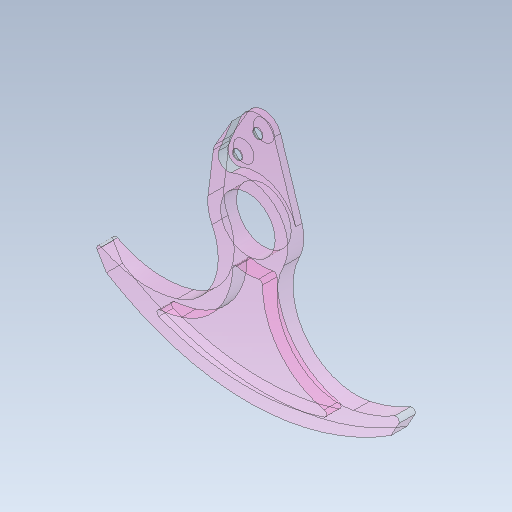
# Autodesk Inventor part: 新型３ヘッケン
Saved by Autodesk Inventor 2020 (Build 240168000, 168)
## iProperties
Created: 2019-03-26
Part Number: 新型３ヘッケン
Material: ポリカーボネート、クリア
Document SubType Name: Modeling
Designer: tanjihayato
Density: 1.2 g/cm^3
Appearance: ポリカーボネート - クリア
Mass: 7.67377 g
Surface Area: 65.6128 cm^2
Volume: 6.39481 cm^3
Author: tanjihayato
Autodesk Inventor part; units mm, degrees
ref_plane "YZ Plane" through (0, 0, 0) normal (1, 0, 0) x (0, 1, 0)
ref_plane "XZ Plane" through (0, 0, 0) normal (0, 1, 0) x (-1, 0, 0)
ref_plane "XY Plane" through (0, 0, 0) normal (0, 0, 1) x (1, 0, 0)
sketch "スケッチ1" plane through (0, 0, 0) normal (0, 0, 1) x (1, 0, 0)
  spline S0 degree 4 poles (44.6679, -57.7205) (44.3779, -57.9011) (43.9715, -58.1517) (43.4481, -58.4698) (42.8069, -58.8523) (42.3406, -59.127) (41.8739, -59.3984) (41.4069, -59.6666) (40.9394, -59.9316) (40.4714, -60.1934) (40.003, -60.452) (39.5341, -60.7075) (39.0646, -60.9598) (38.5946, -61.209) (38.124, -61.455) (37.6528, -61.698) (37.181, -61.9378) (36.7086, -62.1745) (36.2356, -62.4081) (35.7619, -62.6386) (35.2875, -62.8661) (34.8124, -63.0904) (34.3367, -63.3117) (33.8603, -63.5299) (33.3831, -63.745) (32.9053, -63.9571) (32.4267, -64.166) (31.9475, -64.3719) (31.4674, -64.5748) (30.9867, -64.7745) (30.5052, -64.9712) (30.023, -65.1648) (29.54, -65.3554) (29.0563, -65.5428) (28.5719, -65.7272) (28.0867, -65.9085) (27.6008, -66.0867) (27.1141, -66.2618) (26.6267, -66.4339) (26.1386, -66.6028) (25.6497, -66.7686) (25.1602, -66.9313) (24.6699, -67.0909) (24.1789, -67.2474) (23.6872, -67.4008) (23.1948, -67.551) (22.7018, -67.6981) (22.208, -67.8421) (21.7136, -67.983) (21.2185, -68.1207) (20.7227, -68.2552) (20.2264, -68.3866) (19.7293, -68.5148) (19.2317, -68.6399) (18.7335, -68.7617) (18.2346, -68.8805) (17.7352, -68.996) (17.2352, -69.1083) (16.7346, -69.2175) (16.2335, -69.3234) (15.7318, -69.4261) (15.2297, -69.5257) (14.727, -69.622) (14.2238, -69.7151) (13.7202, -69.805) (13.2161, -69.8917) (12.7115, -69.9751) (12.2065, -70.0553) (11.7011, -70.1322) (11.1953, -70.2059) (10.6891, -70.2764) (10.1825, -70.3436) (9.6756, -70.4076) (9.1683, -70.4683) (8.6608, -70.5257) (8.1529, -70.5799) (7.6447, -70.6308) (7.1363, -70.6784) (6.6276, -70.7228) (6.1187, -70.7639) (5.6096, -70.8017) (5.1002, -70.8362) (4.5907, -70.8674) (4.0811, -70.8954) (3.5712, -70.9201) (3.0613, -70.9415) (2.5512, -70.9596) (2.0411, -70.9744) (1.5309, -70.9859) (1.0206, -70.9941) (0.5103, -70.9991) (0, -71.0007) (-0.5103, -70.9991) (-1.0206, -70.9941) (-1.5309, -70.9859) (-2.0411, -70.9744) (-2.5513, -70.9596) (-3.0613, -70.9415) (-3.5712, -70.9201) (-4.0811, -70.8954) (-4.5907, -70.8674) (-5.1003, -70.8362) (-5.6096, -70.8017) (-6.1188, -70.7639) (-6.6277, -70.7228) (-7.1364, -70.6784) (-7.6449, -70.6308) (-8.1531, -70.5799) (-8.661, -70.5257) (-9.1686, -70.4683) (-9.6759, -70.4075) (-10.1829, -70.3436) (-10.6896, -70.2764) (-11.1959, -70.2059) (-11.7018, -70.1322) (-12.2074, -70.0552) (-12.7125, -69.975) (-13.2173, -69.8915) (-13.7216, -69.8049) (-14.2255, -69.7149) (-14.7289, -69.6218) (-15.2318, -69.5254) (-15.7343, -69.4258) (-16.2363, -69.323) (-16.7379, -69.217) (-17.2389, -69.1078) (-17.7394, -68.9954) (-18.2393, -68.8798) (-18.7388, -68.7609) (-19.2377, -68.6389) (-19.736, -68.5137) (-20.2338, -68.3854) (-20.7311, -68.2538) (-21.2277, -68.1191) (-21.7238, -67.9811) (-22.2194, -67.8401) (-22.7144, -67.6958) (-23.2087, -67.5484) (-23.7026, -67.3978) (-24.1958, -67.244) (-24.6885, -67.0871) (-25.1806, -66.927) (-25.6721, -66.7638) (-26.163, -66.5974) (-26.6534, -66.4278) (-27.1433, -66.2551) (-27.6326, -66.0792) (-28.1214, -65.9001) (-28.6097, -65.7179) (-29.0974, -65.5325) (-29.5847, -65.3439) (-30.0715, -65.1521) (-30.5578, -64.9571) (-31.0437, -64.7589) (-31.5292, -64.5576) (-32.0143, -64.3529) (-32.499, -64.1451) (-32.9834, -63.934) (-33.4675, -63.7196) (-33.9513, -63.502) (-34.4349, -63.281) (-34.9183, -63.0567) (-35.4015, -62.8291) (-35.8847, -62.5981) (-36.3678, -62.3637) (-36.8508, -62.1259) (-37.334, -61.8846) (-37.8172, -61.6398) (-38.3007, -61.3914) (-38.7844, -61.1395) (-39.2684, -60.8839) (-39.7528, -60.6247) (-40.2377, -60.3617) (-40.7232, -60.0949) (-41.2094, -59.8243) (-41.6963, -59.5497) (-42.1841, -59.2711) (-42.8575, -58.8816) (-43.4088, -58.5568) (-43.8381, -58.3003) (-44.145, -58.1151) knots 0 0 0 0 0 0.014212 0.019885 0.025551 0.031209 0.036861 0.042507 0.048146 0.053779 0.059407 0.065029 0.070645 0.076257 0.081863 0.087465 0.093062 0.098655 0.104243 0.109828 0.115409 0.120986 0.126559 0.132129 0.137696 0.14326 0.14882 0.154378 0.159933 0.165485 0.171035 0.176582 0.182127 0.187669 0.19321 0.198748 0.204285 0.209819 0.215352 0.220883 0.226412 0.231939 0.237465 0.24299 0.248513 0.254035 0.259556 0.265075 0.270593 0.27611 0.281626 0.287141 0.292655 0.298168 0.30368 0.309191 0.314701 0.320211 0.32572 0.331228 0.336736 0.342242 0.347749 0.353254 0.358759 0.364264 0.369768 0.375272 0.380775 0.386277 0.39178 0.397282 0.402783 0.408284 0.413785 0.419286 0.424786 0.430287 0.435786 0.441286 0.446786 0.452285 0.457784 0.463283 0.468782 0.474281 0.479779 0.485278 0.490776 0.496275 0.501773 0.507272 0.51277 0.518269 0.523767 0.529266 0.534764 0.540263 0.545762 0.551261 0.55676 0.56226 0.567759 0.573259 0.578759 0.584259 0.58976 0.595261 0.600762 0.606263 0.611765 0.617268 0.622771 0.628274 0.633778 0.639282 0.644787 0.650293 0.655799 0.661306 0.666814 0.672322 0.677831 0.683342 0.688853 0.694365 0.699878 0.705392 0.710908 0.716425 0.721943 0.727462 0.732983 0.738505 0.744029 0.749555 0.755082 0.760612 0.766143 0.771677 0.777212 0.78275 0.788291 0.793834 0.79938 0.804928 0.81048 0.816035 0.821593 0.827155 0.832721 0.83829 0.843864 0.849441 0.855024 0.860611 0.866203 0.871801 0.877405 0.883014 0.888629 0.894251 0.89988 0.905517 0.911161 0.916813 0.922473 0.928143 0.933822 0.939511 0.945211 0.950922 0.956645 0.96238 0.968128 0.97389 0.979667 0.985459 1 1 1 1 1
  point P0 (0, 0)
  point P1 (44.2028, -58.0084)
  point P2 (43.7375, -58.293)
  point P3 (43.2719, -58.5742)
  point P4 (42.806, -58.8521)
  point P5 (42.3397, -59.1268)
  point P6 (41.8731, -59.3982)
  point P7 (41.406, -59.6664)
  point P8 (40.9386, -59.9314)
  point P9 (40.4706, -60.1932)
  point P10 (40.0022, -60.4518)
  point P11 (39.5333, -60.7072)
  point P12 (39.0638, -60.9595)
  point P13 (38.5938, -61.2087)
  point P14 (38.1233, -61.4547)
  point P15 (37.6521, -61.6976)
  point P16 (37.1803, -61.9374)
  point P17 (36.7079, -62.1741)
  point P18 (36.2349, -62.4077)
  point P19 (35.7612, -62.6382)
  point P20 (35.2869, -62.8656)
  point P21 (34.8118, -63.09)
  point P22 (34.3361, -63.3112)
  point P23 (33.8597, -63.5294)
  point P24 (33.3826, -63.7445)
  point P25 (32.9048, -63.9566)
  point P26 (32.4262, -64.1656)
  point P27 (31.9469, -64.3714)
  point P28 (31.4669, -64.5743)
  point P29 (30.9862, -64.774)
  point P30 (30.5047, -64.9707)
  point P31 (30.0225, -65.1643)
  point P32 (29.5396, -65.3549)
  point P33 (29.0559, -65.5423)
  point P34 (28.5714, -65.7267)
  point P35 (28.0863, -65.908)
  point P36 (27.6004, -66.0862)
  point P37 (27.1137, -66.2613)
  point P38 (26.6263, -66.4333)
  point P39 (26.1382, -66.6022)
  point P40 (25.6494, -66.768)
  point P41 (25.1598, -66.9307)
  point P42 (24.6696, -67.0903)
  point P43 (24.1786, -67.2468)
  point P44 (23.6869, -67.4002)
  point P45 (23.1945, -67.5504)
  point P46 (22.7014, -67.6975)
  point P47 (22.2077, -67.8415)
  point P48 (21.7133, -67.9824)
  point P49 (21.2182, -68.12)
  point P50 (20.7225, -68.2546)
  point P51 (20.2261, -68.386)
  point P52 (19.7291, -68.5142)
  point P53 (19.2315, -68.6392)
  point P54 (18.7332, -68.7611)
  point P55 (18.2344, -68.8798)
  point P56 (17.735, -68.9953)
  point P57 (17.235, -69.1077)
  point P58 (16.7344, -69.2168)
  point P59 (16.2333, -69.3228)
  point P60 (15.7317, -69.4255)
  point P61 (15.2295, -69.525)
  point P62 (14.7268, -69.6214)
  point P63 (14.2237, -69.7145)
  point P64 (13.72, -69.8043)
  point P65 (13.2159, -69.891)
  point P66 (12.7113, -69.9744)
  point P67 (12.2064, -70.0546)
  point P68 (11.701, -70.1316)
  point P69 (11.1952, -70.2053)
  point P70 (10.689, -70.2757)
  point P71 (10.1824, -70.3429)
  point P72 (9.6755, -70.4069)
  point P73 (9.1682, -70.4676)
  point P74 (8.6607, -70.525)
  point P75 (8.1528, -70.5792)
  point P76 (7.6446, -70.6301)
  point P77 (7.1362, -70.6777)
  point P78 (6.6275, -70.7221)
  point P79 (6.1186, -70.7632)
  point P80 (5.6095, -70.801)
  point P81 (5.1002, -70.8355)
  point P82 (4.5907, -70.8668)
  point P83 (4.081, -70.8947)
  point P84 (3.5712, -70.9194)
  point P85 (3.0613, -70.9408)
  point P86 (2.5512, -70.9589)
  point P87 (2.0411, -70.9737)
  point P88 (1.5309, -70.9852)
  point P89 (1.0206, -70.9934)
  point P90 (0.5103, -70.9984)
  point P91 (0, -71)
  point P92 (-0.5103, -70.9984)
  point P93 (-1.0206, -70.9934)
  point P94 (-1.5309, -70.9852)
  point P95 (-2.0411, -70.9737)
  point P96 (-2.5512, -70.9589)
  point P97 (-3.0613, -70.9408)
  point P98 (-3.5712, -70.9194)
  point P99 (-4.081, -70.8947)
  point P100 (-4.5907, -70.8668)
  point P101 (-5.1002, -70.8355)
  point P102 (-5.6095, -70.801)
  point P103 (-6.1187, -70.7632)
  point P104 (-6.6276, -70.7221)
  point P105 (-7.1363, -70.6777)
  point P106 (-7.6448, -70.6301)
  point P107 (-8.153, -70.5792)
  point P108 (-8.6609, -70.525)
  point P109 (-9.1685, -70.4676)
  point P110 (-9.6758, -70.4069)
  point P111 (-10.1828, -70.3429)
  point P112 (-10.6894, -70.2757)
  point P113 (-11.1957, -70.2052)
  point P114 (-11.7017, -70.1315)
  point P115 (-12.2072, -70.0545)
  point P116 (-12.7124, -69.9743)
  point P117 (-13.2171, -69.8909)
  point P118 (-13.7214, -69.8042)
  point P119 (-14.2253, -69.7143)
  point P120 (-14.7287, -69.6211)
  point P121 (-15.2316, -69.5248)
  point P122 (-15.7341, -69.4252)
  point P123 (-16.2361, -69.3224)
  point P124 (-16.7376, -69.2164)
  point P125 (-17.2386, -69.1072)
  point P126 (-17.7391, -68.9948)
  point P127 (-18.2391, -68.8791)
  point P128 (-18.7385, -68.7603)
  point P129 (-19.2374, -68.6383)
  point P130 (-19.7357, -68.5131)
  point P131 (-20.2335, -68.3847)
  point P132 (-20.7307, -68.2532)
  point P133 (-21.2274, -68.1184)
  point P134 (-21.7235, -67.9805)
  point P135 (-22.219, -67.8395)
  point P136 (-22.714, -67.6952)
  point P137 (-23.2084, -67.5478)
  point P138 (-23.7022, -67.3972)
  point P139 (-24.1954, -67.2435)
  point P140 (-24.688, -67.0865)
  point P141 (-25.1801, -66.9265)
  point P142 (-25.6716, -66.7632)
  point P143 (-26.1626, -66.5968)
  point P144 (-26.653, -66.4273)
  point P145 (-27.1428, -66.2546)
  point P146 (-27.6321, -66.0787)
  point P147 (-28.1209, -65.8996)
  point P148 (-28.6091, -65.7174)
  point P149 (-29.0968, -65.532)
  point P150 (-29.5841, -65.3434)
  point P151 (-30.0709, -65.1516)
  point P152 (-30.5572, -64.9567)
  point P153 (-31.043, -64.7585)
  point P154 (-31.5285, -64.5571)
  point P155 (-32.0136, -64.3525)
  point P156 (-32.4983, -64.1447)
  point P157 (-32.9826, -63.9336)
  point P158 (-33.4667, -63.7192)
  point P159 (-33.9505, -63.5016)
  point P160 (-34.434, -63.2807)
  point P161 (-34.9174, -63.0564)
  point P162 (-35.4006, -62.8288)
  point P163 (-35.8837, -62.5978)
  point P164 (-36.3668, -62.3635)
  point P165 (-36.8498, -62.1257)
  point P166 (-37.3329, -61.8844)
  point P167 (-37.8161, -61.6396)
  point P168 (-38.2995, -61.3913)
  point P169 (-38.7831, -61.1394)
  point P170 (-39.2671, -60.8839)
  point P171 (-39.7515, -60.6247)
  point P172 (-40.2363, -60.3617)
  point P173 (-40.7217, -60.095)
  point P174 (-41.2079, -59.8244)
  point P175 (-41.6947, -59.5498)
  point P176 (-42.1825, -59.2713)
  point P177 (-42.6713, -58.9886)
  point P178 (-43.1612, -58.7017)
  point P179 (-43.6524, -58.4106)
  constraints: 181 other
sketch "スケッチ2" plane through (0, 0, 0) normal (0, 0, 1) x (1, 0, 0)
  spline S0 degree 4 poles (44.6679, -57.7205) (44.3779, -57.9011) (43.9715, -58.1517) (43.4481, -58.4698) (42.8069, -58.8523) (42.3406, -59.127) (41.8739, -59.3984) (41.4069, -59.6666) (40.9394, -59.9316) (40.4714, -60.1934) (40.003, -60.452) (39.5341, -60.7075) (39.0646, -60.9598) (38.5946, -61.209) (38.124, -61.455) (37.6528, -61.698) (37.181, -61.9378) (36.7086, -62.1745) (36.2356, -62.4081) (35.7619, -62.6386) (35.2875, -62.8661) (34.8124, -63.0904) (34.3367, -63.3117) (33.8603, -63.5299) (33.3831, -63.745) (32.9053, -63.9571) (32.4267, -64.166) (31.9475, -64.3719) (31.4674, -64.5748) (30.9867, -64.7745) (30.5052, -64.9712) (30.023, -65.1648) (29.54, -65.3554) (29.0563, -65.5428) (28.5719, -65.7272) (28.0867, -65.9085) (27.6008, -66.0867) (27.1141, -66.2618) (26.6267, -66.4339) (26.1386, -66.6028) (25.6497, -66.7686) (25.1602, -66.9313) (24.6699, -67.0909) (24.1789, -67.2474) (23.6872, -67.4008) (23.1948, -67.551) (22.7018, -67.6981) (22.208, -67.8421) (21.7136, -67.983) (21.2185, -68.1207) (20.7227, -68.2552) (20.2264, -68.3866) (19.7293, -68.5148) (19.2317, -68.6399) (18.7335, -68.7617) (18.2346, -68.8805) (17.7352, -68.996) (17.2352, -69.1083) (16.7346, -69.2175) (16.2335, -69.3234) (15.7318, -69.4261) (15.2297, -69.5257) (14.727, -69.622) (14.2238, -69.7151) (13.7202, -69.805) (13.2161, -69.8917) (12.7115, -69.9751) (12.2065, -70.0553) (11.7011, -70.1322) (11.1953, -70.2059) (10.6891, -70.2764) (10.1825, -70.3436) (9.6756, -70.4076) (9.1683, -70.4683) (8.6608, -70.5257) (8.1529, -70.5799) (7.6447, -70.6308) (7.1363, -70.6784) (6.6276, -70.7228) (6.1187, -70.7639) (5.6096, -70.8017) (5.1002, -70.8362) (4.5907, -70.8674) (4.0811, -70.8954) (3.5712, -70.9201) (3.0613, -70.9415) (2.5512, -70.9596) (2.0411, -70.9744) (1.5309, -70.9859) (1.0206, -70.9941) (0.5103, -70.9991) (0, -71.0007) (-0.5103, -70.9991) (-1.0206, -70.9941) (-1.5309, -70.9859) (-2.0411, -70.9744) (-2.5513, -70.9596) (-3.0613, -70.9415) (-3.5712, -70.9201) (-4.0811, -70.8954) (-4.5907, -70.8674) (-5.1003, -70.8362) (-5.6096, -70.8017) (-6.1188, -70.7639) (-6.6277, -70.7228) (-7.1364, -70.6784) (-7.6449, -70.6308) (-8.1531, -70.5799) (-8.661, -70.5257) (-9.1686, -70.4683) (-9.6759, -70.4075) (-10.1829, -70.3436) (-10.6896, -70.2764) (-11.1959, -70.2059) (-11.7018, -70.1322) (-12.2074, -70.0552) (-12.7125, -69.975) (-13.2173, -69.8915) (-13.7216, -69.8049) (-14.2255, -69.7149) (-14.7289, -69.6218) (-15.2318, -69.5254) (-15.7343, -69.4258) (-16.2363, -69.323) (-16.7379, -69.217) (-17.2389, -69.1078) (-17.7394, -68.9954) (-18.2393, -68.8798) (-18.7388, -68.7609) (-19.2377, -68.6389) (-19.736, -68.5137) (-20.2338, -68.3854) (-20.7311, -68.2538) (-21.2277, -68.1191) (-21.7238, -67.9811) (-22.2194, -67.8401) (-22.7144, -67.6958) (-23.2087, -67.5484) (-23.7026, -67.3978) (-24.1958, -67.244) (-24.6885, -67.0871) (-25.1806, -66.927) (-25.6721, -66.7638) (-26.163, -66.5974) (-26.6534, -66.4278) (-27.1433, -66.2551) (-27.6326, -66.0792) (-28.1214, -65.9001) (-28.6097, -65.7179) (-29.0974, -65.5325) (-29.5847, -65.3439) (-30.0715, -65.1521) (-30.5578, -64.9571) (-31.0437, -64.7589) (-31.5292, -64.5576) (-32.0143, -64.3529) (-32.499, -64.1451) (-32.9834, -63.934) (-33.4675, -63.7196) (-33.9513, -63.502) (-34.4349, -63.281) (-34.9183, -63.0567) (-35.4015, -62.8291) (-35.8847, -62.5981) (-36.3678, -62.3637) (-36.8508, -62.1259) (-37.334, -61.8846) (-37.8172, -61.6398) (-38.3007, -61.3914) (-38.7844, -61.1395) (-39.2684, -60.8839) (-39.7528, -60.6247) (-40.2377, -60.3617) (-40.7232, -60.0949) (-41.2094, -59.8243) (-41.6963, -59.5497) (-42.1841, -59.2711) (-42.8575, -58.8816) (-43.4088, -58.5568) (-43.8381, -58.3003) (-44.145, -58.1151) knots 0 0 0 0 0 0.014212 0.019885 0.025551 0.031209 0.036861 0.042507 0.048146 0.053779 0.059407 0.065029 0.070645 0.076257 0.081863 0.087465 0.093062 0.098655 0.104243 0.109828 0.115409 0.120986 0.126559 0.132129 0.137696 0.14326 0.14882 0.154378 0.159933 0.165485 0.171035 0.176582 0.182127 0.187669 0.19321 0.198748 0.204285 0.209819 0.215352 0.220883 0.226412 0.231939 0.237465 0.24299 0.248513 0.254035 0.259556 0.265075 0.270593 0.27611 0.281626 0.287141 0.292655 0.298168 0.30368 0.309191 0.314701 0.320211 0.32572 0.331228 0.336736 0.342242 0.347749 0.353254 0.358759 0.364264 0.369768 0.375272 0.380775 0.386277 0.39178 0.397282 0.402783 0.408284 0.413785 0.419286 0.424786 0.430287 0.435786 0.441286 0.446786 0.452285 0.457784 0.463283 0.468782 0.474281 0.479779 0.485278 0.490776 0.496275 0.501773 0.507272 0.51277 0.518269 0.523767 0.529266 0.534764 0.540263 0.545762 0.551261 0.55676 0.56226 0.567759 0.573259 0.578759 0.584259 0.58976 0.595261 0.600762 0.606263 0.611765 0.617268 0.622771 0.628274 0.633778 0.639282 0.644787 0.650293 0.655799 0.661306 0.666814 0.672322 0.677831 0.683342 0.688853 0.694365 0.699878 0.705392 0.710908 0.716425 0.721943 0.727462 0.732983 0.738505 0.744029 0.749555 0.755082 0.760612 0.766143 0.771677 0.777212 0.78275 0.788291 0.793834 0.79938 0.804928 0.81048 0.816035 0.821593 0.827155 0.832721 0.83829 0.843864 0.849441 0.855024 0.860611 0.866203 0.871801 0.877405 0.883014 0.888629 0.894251 0.89988 0.905517 0.911161 0.916813 0.922473 0.928143 0.933822 0.939511 0.945211 0.950922 0.956645 0.96238 0.968128 0.97389 0.979667 0.985459 1 1 1 1 1 projected
  circle A0 centre (0, 0) radius 1.5
  circle A1 centre (0, -23) radius 8.525
  line L0 (0, 0) -> (0, -23) construction
  circle A2 centre (0, -23) radius 12.525
  circle A3 centre (0, 0) radius 5.5
  line L1 (-5.2372, 1.6799) -> (-11.9265, -19.1744)
  line L2 (5.2372, 1.6799) -> (11.9265, -19.1744)
  line L3 (-44.145, -58.1151) -> (-49.1112, -49.8307)
  line L4 (44.6679, -57.7205) -> (48.9949, -49.8307)
  arc A4 (-22.0046, -54.1258) -> (-11.1841, -28.6384) centre (-27.3796, -36.8033) ccw
  arc A5 (11.1932, -28.6204) -> (33.009, -56.7784) centre (28.8377, -37.4801) ccw
  arc A6 (-49.1112, -49.8307) -> (-22.0046, -54.1258) centre (-31.2017, -24.4856) ccw
  arc A7 (33.009, -56.7784) -> (48.9949, -49.8307) centre (23.6069, -13.28) ccw
  dimension "d0" = 3
  dimension "d1" = 17.05
  dimension "d2" = 23
  dimension "d3" = 4
  dimension "d4" = 4
  constraints: 14 point on circle, 10 end point, 8 centre point, 8 tangent, 1 coincident, 1 vertical
  measures "d0" diameter of A0
  measures "d1" diameter of A1
  measures "d2" distance of L0.start L0.end
  measures "d3" radial gap between concentric circles of A1 A2
  measures "d4" radial gap between concentric circles of A0 A3
extrude "押し出し1" add sketch "スケッチ2" along normal blind 5
sketch "スケッチ3" plane through (0, 0, 5) normal (0, 0, 1) x (1, 0, 0)
  circle A0 centre (0, -23) radius 8.525 projected
  circle A1 centre (0, 0) radius 1.5 projected
  arc A2 (5.2372, 1.6799) -> (-5.2372, 1.6799) centre (0, 0) ccw projected
  line L0 (-5.2372, 1.6799) -> (-11.9265, -19.1744) projected
  arc A3 (-11.9265, -19.1744) -> (-11.1841, -28.6384) centre (0, -23) ccw projected
  arc A4 (-11.1841, -28.6384) -> (-22.0046, -54.1258) centre (-27.3796, -36.8033) ccw projected
  arc A5 (-22.0046, -54.1258) -> (-49.1112, -49.8307) centre (-31.2017, -24.4856) ccw projected
  spline S0 degree 4 poles (-44.145, -58.1151) (-43.8381, -58.3003) (-43.4088, -58.5568) (-42.8575, -58.8816) (-42.1841, -59.2711) (-41.6963, -59.5497) (-41.2094, -59.8243) (-40.7232, -60.0949) (-40.2377, -60.3617) (-39.7528, -60.6247) (-39.2684, -60.8839) (-38.7844, -61.1395) (-38.3007, -61.3914) (-37.8172, -61.6398) (-37.334, -61.8846) (-36.8508, -62.1259) (-36.3678, -62.3637) (-35.8847, -62.5981) (-35.4015, -62.8291) (-34.9183, -63.0567) (-34.4349, -63.281) (-33.9513, -63.502) (-33.4675, -63.7196) (-32.9834, -63.934) (-32.499, -64.1451) (-32.0143, -64.3529) (-31.5292, -64.5576) (-31.0437, -64.7589) (-30.5578, -64.9571) (-30.0715, -65.1521) (-29.5847, -65.3439) (-29.0974, -65.5325) (-28.6097, -65.7179) (-28.1214, -65.9001) (-27.6326, -66.0792) (-27.1433, -66.2551) (-26.6534, -66.4278) (-26.163, -66.5974) (-25.6721, -66.7638) (-25.1806, -66.927) (-24.6885, -67.0871) (-24.1958, -67.244) (-23.7026, -67.3978) (-23.2087, -67.5484) (-22.7144, -67.6958) (-22.2194, -67.8401) (-21.7238, -67.9811) (-21.2277, -68.1191) (-20.7311, -68.2538) (-20.2338, -68.3854) (-19.736, -68.5137) (-19.2377, -68.6389) (-18.7388, -68.7609) (-18.2393, -68.8798) (-17.7394, -68.9954) (-17.2389, -69.1078) (-16.7379, -69.217) (-16.2363, -69.323) (-15.7343, -69.4258) (-15.2318, -69.5254) (-14.7289, -69.6218) (-14.2255, -69.7149) (-13.7216, -69.8049) (-13.2173, -69.8915) (-12.7125, -69.975) (-12.2074, -70.0552) (-11.7018, -70.1322) (-11.1959, -70.2059) (-10.6896, -70.2764) (-10.1829, -70.3436) (-9.6759, -70.4075) (-9.1686, -70.4683) (-8.661, -70.5257) (-8.1531, -70.5799) (-7.6449, -70.6308) (-7.1364, -70.6784) (-6.6277, -70.7228) (-6.1188, -70.7639) (-5.6096, -70.8017) (-5.1003, -70.8362) (-4.5907, -70.8674) (-4.0811, -70.8954) (-3.5712, -70.9201) (-3.0613, -70.9415) (-2.5513, -70.9596) (-2.0411, -70.9744) (-1.5309, -70.9859) (-1.0206, -70.9941) (-0.5103, -70.9991) (0, -71.0007) (0.5103, -70.9991) (1.0206, -70.9941) (1.5309, -70.9859) (2.0411, -70.9744) (2.5512, -70.9596) (3.0613, -70.9415) (3.5712, -70.9201) (4.0811, -70.8954) (4.5907, -70.8674) (5.1002, -70.8362) (5.6096, -70.8017) (6.1187, -70.7639) (6.6276, -70.7228) (7.1363, -70.6784) (7.6447, -70.6308) (8.1529, -70.5799) (8.6608, -70.5257) (9.1683, -70.4683) (9.6756, -70.4076) (10.1825, -70.3436) (10.6891, -70.2764) (11.1953, -70.2059) (11.7011, -70.1322) (12.2065, -70.0553) (12.7115, -69.9751) (13.2161, -69.8917) (13.7202, -69.805) (14.2238, -69.7151) (14.727, -69.622) (15.2297, -69.5257) (15.7318, -69.4261) (16.2335, -69.3234) (16.7346, -69.2175) (17.2352, -69.1083) (17.7352, -68.996) (18.2346, -68.8805) (18.7335, -68.7617) (19.2317, -68.6399) (19.7293, -68.5148) (20.2264, -68.3866) (20.7227, -68.2552) (21.2185, -68.1207) (21.7136, -67.983) (22.208, -67.8421) (22.7018, -67.6981) (23.1948, -67.551) (23.6872, -67.4008) (24.1789, -67.2474) (24.6699, -67.0909) (25.1602, -66.9313) (25.6497, -66.7686) (26.1386, -66.6028) (26.6267, -66.4339) (27.1141, -66.2618) (27.6008, -66.0867) (28.0867, -65.9085) (28.5719, -65.7272) (29.0563, -65.5428) (29.54, -65.3554) (30.023, -65.1648) (30.5052, -64.9712) (30.9867, -64.7745) (31.4674, -64.5748) (31.9475, -64.3719) (32.4267, -64.166) (32.9053, -63.9571) (33.3831, -63.745) (33.8603, -63.5299) (34.3367, -63.3117) (34.8124, -63.0904) (35.2875, -62.8661) (35.7619, -62.6386) (36.2356, -62.4081) (36.7086, -62.1745) (37.181, -61.9378) (37.6528, -61.698) (38.124, -61.455) (38.5946, -61.209) (39.0646, -60.9598) (39.5341, -60.7075) (40.003, -60.452) (40.4714, -60.1934) (40.9394, -59.9316) (41.4069, -59.6666) (41.8739, -59.3984) (42.3406, -59.127) (42.8069, -58.8523) (43.4481, -58.4698) (43.9715, -58.1517) (44.3779, -57.9011) (44.6679, -57.7205) knots 0 0 0 0 0 0.014541 0.020333 0.02611 0.031872 0.03762 0.043355 0.049078 0.054789 0.060489 0.066178 0.071857 0.077527 0.083187 0.088839 0.094483 0.10012 0.105749 0.111371 0.116986 0.122595 0.128199 0.133797 0.139389 0.144976 0.150559 0.156136 0.16171 0.167279 0.172845 0.178407 0.183965 0.18952 0.195072 0.20062 0.206166 0.211709 0.21725 0.222788 0.228323 0.233857 0.239388 0.244918 0.250445 0.255971 0.261495 0.267017 0.272538 0.278057 0.283575 0.289092 0.294608 0.300122 0.305635 0.311147 0.316658 0.322169 0.327678 0.333186 0.338694 0.344201 0.349707 0.355213 0.360718 0.366222 0.371726 0.377229 0.382732 0.388235 0.393737 0.399238 0.404739 0.41024 0.415741 0.421241 0.426741 0.432241 0.43774 0.44324 0.448739 0.454238 0.459737 0.465236 0.470734 0.476233 0.481731 0.48723 0.492728 0.498227 0.503725 0.509224 0.514722 0.520221 0.525719 0.531218 0.536717 0.542216 0.547715 0.553214 0.558714 0.564214 0.569713 0.575214 0.580714 0.586215 0.591716 0.597217 0.602718 0.60822 0.613723 0.619225 0.624728 0.630232 0.635736 0.641241 0.646746 0.652251 0.657758 0.663264 0.668772 0.67428 0.679789 0.685299 0.690809 0.69632 0.701832 0.707345 0.712859 0.718374 0.72389 0.729407 0.734925 0.740444 0.745965 0.751487 0.75701 0.762535 0.768061 0.773588 0.779117 0.784648 0.790181 0.795715 0.801252 0.80679 0.812331 0.817873 0.823418 0.828965 0.834515 0.840067 0.845622 0.85118 0.85674 0.862304 0.867871 0.873441 0.879014 0.884591 0.890172 0.895757 0.901345 0.906938 0.912535 0.918137 0.923743 0.929355 0.934971 0.940593 0.946221 0.951854 0.957493 0.963139 0.968791 0.974449 0.980115 0.985788 1 1 1 1 1 projected
  arc A6 (48.9949, -49.8307) -> (33.009, -56.7784) centre (23.6069, -13.28) ccw projected
  arc A7 (33.009, -56.7784) -> (11.1932, -28.6204) centre (28.8377, -37.4801) ccw projected
  arc A8 (11.1932, -28.6204) -> (11.9265, -19.1744) centre (0, -23) ccw projected
  line L1 (11.9265, -19.1744) -> (5.2372, 1.6799) projected
  arc A9 (33.8541, -60.6881) -> (51.2768, -53.116) centre (23.6069, -13.28) ccw
  arc A10 (4.6594, -35.6971) -> (27.888, -61.7054) centre (28.8377, -37.4801) ccw
  arc A11 (7.6185, -26.8254) -> (8.1176, -20.3962) centre (0, -23) ccw
  line L2 (8.1176, -20.3962) -> (1.4283, 0.4582)
  arc A12 (1.4283, 0.4582) -> (-1.4283, 0.4582) centre (0, 0) ccw
  line L3 (-1.4283, 0.4582) -> (-8.1176, -20.3962)
  arc A13 (-8.1176, -20.3962) -> (-7.6123, -26.8377) centre (0, -23) ccw
  arc A14 (-20.671, -58.4236) -> (-4.7715, -35.6554) centre (-27.3796, -36.8033) ccw
  arc A15 (-31.9588, -60.0118) -> (-20.671, -58.4236) centre (-31.2017, -24.4856) ccw
  arc A16 (-4.7715, -35.6554) -> (4.6594, -35.6971) centre (0, -23) ccw
  spline S1 degree 5 poles (-31.9588, -60.0118) (-25.8706, -62.7405) (-19.5197, -64.8823) (-12.9481, -66.3291) (-0.6399, -67.6295) (11.6561, -66.4119) (17.215, -65.3274) (22.6392, -63.7424) (27.888, -61.7054) knots 0 0 0 0 0 0 0.542327 0.542327 0.542327 1 1 1 1 1 1
  dimension "d7" = 4
  dimension "d8" = 4.5
  dimension "d10" = 5
  dimension "d11" = 4.5
  dimension "d12" = 4.5
  constraints: 17 centre point, 16 point on circle, 4 end point, 1 coincident, 9 other
  measures "d8" radial gap between concentric circles of A7 A10
  measures "d10" radial gap between concentric circles of A16 A0
  measures "d11" radial gap between concentric circles of A4 A14
  measures "d12" radial gap between concentric circles of A5 A15
extrude "押し出し2" cut sketch "スケッチ3" against normal blind 4.5 contours A16 A10 A6 A14 A5 | A5 A14 A16 | A6 A10 S1 A15 A14
fillet "フィレット1" radius 1 4 edges at (4.6594, -35.6971, 2.75) (-4.7715, -35.6554, 2.75) (27.888, -61.7054, 2.75) (-31.9588, -60.0118, 2.75)
sketch "スケッチ4" plane through (0, 0, 5) normal (0, 0, 1) x (1, 0, 0)
  arc A0 (4.5969, -37.0887) -> (23.8174, -61.1986) centre (28.8377, -37.4801) ccw projected
  arc A1 (-27.5161, -59.8282) -> (-20.671, -58.4236) centre (-31.2017, -24.4856) ccw projected
  arc A2 (-20.671, -58.4236) -> (-4.7434, -37.0245) centre (-27.3796, -36.8033) ccw projected
  arc A3 (-3.4858, -36.0681) -> (-4.7434, -37.0245) centre (-3.7435, -37.0343) ccw projected
  arc A4 (-3.4858, -36.0681) -> (3.3494, -36.1037) centre (0, -23) ccw projected
  arc A5 (4.5969, -37.0887) -> (3.3494, -36.1037) centre (3.597, -37.0726) ccw projected
  circle A6 centre (0, -23) radius 8.525 projected
  circle A7 centre (0, 0) radius 1.5 projected
  arc A8 (5.2372, 1.6799) -> (-5.2372, 1.6799) centre (0, 0) ccw projected
  line L0 (-5.2372, 1.6799) -> (-11.9265, -19.1744) projected
  arc A9 (-11.9265, -19.1744) -> (-11.1841, -28.6384) centre (0, -23) ccw projected
  arc A10 (-22.0046, -54.1258) -> (-11.1841, -28.6384) centre (-27.3796, -36.8033) ccw projected
  arc A11 (-49.1112, -49.8307) -> (-22.0046, -54.1258) centre (-31.2017, -24.4856) ccw projected
  line L1 (-49.1112, -49.8307) -> (-44.145, -58.1151) projected
  line L2 (44.6679, -57.7205) -> (48.9949, -49.8307) projected
  arc A12 (33.009, -56.7784) -> (48.9949, -49.8307) centre (23.6069, -13.28) ccw projected
  arc A13 (11.1932, -28.6204) -> (33.009, -56.7784) centre (28.8377, -37.4801) ccw projected
  arc A14 (11.1932, -28.6204) -> (11.9265, -19.1744) centre (0, -23) ccw projected
  line L3 (11.9265, -19.1744) -> (5.2372, 1.6799) projected
  arc A15 (11.9265, -19.1744) -> (-11.9265, -19.1744) centre (0, -23) ccw
  dimension "d16" = 12.525
  constraints: 2 point on circle, 2 point on line, 1 centre point, 1 coincident, 4 other
  measures "d16" radius of A15
extrude "押し出し3" cut sketch "スケッチ4" against normal blind 3 contours L3 A15 L0 A8
sketch "スケッチ5" plane through (0, 0, 2) normal (0, 0, 1) x (1, 0, 0)
  circle A0 centre (0, 0) radius 1.5 projected
  line L0 (5.2372, 1.6799) -> (11.9265, -19.1744) projected
  arc A1 (5.2372, 1.6799) -> (-5.2372, 1.6799) centre (0, 0) ccw projected
  line L1 (-11.9265, -19.1744) -> (-5.2372, 1.6799) projected
  arc A2 (11.9265, -19.1744) -> (-11.9265, -19.1744) centre (0, -23) ccw projected
  circle A3 centre (-6.3066, -8.8137) radius 1.5
  arc A4 (-10.1922, -6.5439) -> (-10.7715, -8.253) centre (-6.3066, -8.8137) ccw
  circle A5 centre (-6.3066, -8.8137) radius 4.5
  arc A6 (11.1932, -28.6204) -> (-11.1841, -28.6384) centre (0, -23) ccw projected
  line L2 (-12.4274, -21.4394) -> (-10.7715, -8.253)
  line L3 (-10.1922, -6.5439) -> (-4.7491, 2.7742)
  arc A7 (5.2372, 1.6799) -> (-5.2372, 1.6799) centre (0, 0) ccw projected
  line L4 (0, 0) -> (-6.3066, -8.8137)
  line L5 (-6.3066, -8.8137) -> (0, -23)
  dimension "d20" = 3
  dimension "d22" = 9
  constraints: 8 end point, 4 point on circle, 4 tangent, 3 centre point, 1 coincident, 1 concentric, 2 other
  measures "d20" diameter of A3
  measures "d22" diameter of A5
extrude "押し出し4" add sketch "スケッチ5" against normal blind 2 contours A0 | L0 A2 A5 L1 A1 | A1 L1 A5 L3 | A2 L5 A3 L4 A5 | A5 L1 A4 | A2 A5 L1 L4 A3 L5 | A5 L1 A6 L2 | A2 L1 A5 | L5 L4 A3 | A3 L4 L5
extrude "押し出し5" cut sketch "スケッチ5" against normal blind 2 contours A0 | L5 L4 A3 | A3 L4 L5
fillet "フィレット2" radius 1 2 edges at (-49.1112, -49.8307, 2.5) (48.9949, -49.8307, 2.5)
sketch "スケッチ6" plane through (0, 0, 5) normal (0, 0, 1) x (1, 0, 0)
  arc A0 (47.1325, -53.2266) -> (45.758, -51.8784) centre (46.2557, -52.7457) ccw projected
  arc A1 (33.009, -56.7784) -> (45.758, -51.8784) centre (23.6069, -13.28) ccw projected
  arc A2 (11.1932, -28.6204) -> (33.009, -56.7784) centre (28.8377, -37.4801) ccw projected
  arc A3 (11.1932, -28.6204) -> (-11.1841, -28.6384) centre (0, -23) ccw projected
  arc A4 (-22.0046, -54.1258) -> (-11.1841, -28.6384) centre (-27.3796, -36.8033) ccw projected
  arc A5 (-45.6895, -51.9306) -> (-22.0046, -54.1258) centre (-31.2017, -24.4856) ccw projected
  arc A6 (-45.6895, -51.9306) -> (-47.014, -53.3291) centre (-46.1563, -52.815) ccw projected
  line L0 (-47.014, -53.3291) -> (-44.145, -58.1151) projected
  line L1 (44.6679, -57.7205) -> (47.1325, -53.2266) projected
  arc A7 (4.5969, -37.0887) -> (23.8174, -61.1986) centre (28.8377, -37.4801) ccw projected
  arc A8 (-27.5161, -59.8282) -> (-20.671, -58.4236) centre (-31.2017, -24.4856) ccw projected
  arc A9 (-20.671, -58.4236) -> (-4.7434, -37.0245) centre (-27.3796, -36.8033) ccw projected
  arc A10 (-3.4858, -36.0681) -> (-4.7434, -37.0245) centre (-3.7435, -37.0343) ccw projected
  arc A11 (-3.4858, -36.0681) -> (3.3494, -36.1037) centre (0, -23) ccw projected
  arc A12 (4.5969, -37.0887) -> (3.3494, -36.1037) centre (3.597, -37.0726) ccw projected
  circle A13 centre (0, -23) radius 8.525 projected
  circle A14 centre (0, 0) radius 1.5 projected
  circle A15 centre (-6.3066, -8.8137) radius 1.5 projected
  line L2 (5.2372, 1.6799) -> (11.9265, -19.1744) projected
  arc A16 (5.2372, 1.6799) -> (-4.7491, 2.7742) centre (0, 0) ccw projected
  line L3 (-4.7491, 2.7742) -> (-10.1922, -6.5439) projected
  arc A17 (-10.1922, -6.5439) -> (-10.7715, -8.253) centre (-6.3066, -8.8137) ccw projected
  line L4 (-10.7715, -8.253) -> (-12.4274, -21.4394) projected
  arc A18 (11.9265, -19.1744) -> (-12.4274, -21.4394) centre (0, -23) ccw projected
  arc A19 (-9.0832, -7.6778) -> (-5.0879, -11.555) centre (-6.3066, -8.8137) ccw
  line L5 (-9.0832, -7.6778) -> (-4.9441, 2.4403)
  constraints: 3 point on circle, 3 tangent, 2 end point, 1 centre point, 1 coincident, 1 point on line, 4 other
extrude "押し出し6" add sketch "スケッチ6" against normal blind 3 contours A3 L4 A17 L3 L5 A19
sketch "スケッチ7" plane through (0, 0, 2) normal (0, 0, 1) x (1, 0, 0)
  arc A0 (-9.0832, -7.6778) -> (-5.0879, -11.555) centre (-6.3066, -8.8137) ccw
  arc A1 (11.9265, -19.1744) -> (-5.0879, -11.555) centre (0, -23) ccw
  line L0 (5.2372, 1.6799) -> (11.9265, -19.1744)
  arc A2 (5.2372, 1.6799) -> (-4.7491, 2.7742) centre (0, 0) ccw
  line L1 (-4.7491, 2.7742) -> (-4.9441, 2.4403)
  circle A3 centre (-6.3066, -8.8137) radius 1.5
  circle A4 centre (0, 0) radius 1.5
  line L2 (7.036, 2.62) -> (13.8309, -18.5636)
  line L3 (5.2372, 1.6799) -> (11.9265, -19.1744)
  arc A5 (11.9265, -19.1744) -> (13.8309, -18.5636) centre (12.8787, -18.869) ccw
  arc A6 (7.1416, 2.2908) -> (-7.0919, 2.4404) centre (0, 0) ccw
  line L4 (-7.0919, 2.4404) -> (-10.7715, -8.253)
  arc A7 (45.758, -51.8784) -> (47.1325, -53.2266) centre (46.2557, -52.7457) ccw
  arc A8 (45.758, -51.8784) -> (33.009, -56.7784) centre (23.6069, -13.28) ccw
  arc A9 (33.009, -56.7784) -> (11.1932, -28.6204) centre (28.8377, -37.4801) ccw
  arc A10 (11.1932, -28.6204) -> (11.9265, -19.1744) centre (0, -23) ccw
  line L5 (-10.7715, -8.253) -> (-12.4274, -21.4394)
  arc A11 (-12.4274, -21.4394) -> (-11.1841, -28.6384) centre (0, -23) ccw
  arc A12 (-11.1841, -28.6384) -> (-22.0046, -54.1258) centre (-27.3796, -36.8033) ccw
  arc A13 (-22.0046, -54.1258) -> (-45.6895, -51.9306) centre (-31.2017, -24.4856) ccw
  arc A14 (-47.014, -53.3291) -> (-45.6895, -51.9306) centre (-46.1563, -52.815) ccw
  line L6 (-47.014, -53.3291) -> (-44.145, -58.1151)
  spline S0 degree 4 poles (-44.145, -58.1151) (-43.8381, -58.3003) (-43.4088, -58.5568) (-42.8575, -58.8816) (-42.1841, -59.2711) (-41.6963, -59.5497) (-41.2094, -59.8243) (-40.7232, -60.0949) (-40.2377, -60.3617) (-39.7528, -60.6247) (-39.2684, -60.8839) (-38.7844, -61.1395) (-38.3007, -61.3914) (-37.8172, -61.6398) (-37.334, -61.8846) (-36.8508, -62.1259) (-36.3678, -62.3637) (-35.8847, -62.5981) (-35.4015, -62.8291) (-34.9183, -63.0567) (-34.4349, -63.281) (-33.9513, -63.502) (-33.4675, -63.7196) (-32.9834, -63.934) (-32.499, -64.1451) (-32.0143, -64.3529) (-31.5292, -64.5576) (-31.0437, -64.7589) (-30.5578, -64.9571) (-30.0715, -65.1521) (-29.5847, -65.3439) (-29.0974, -65.5325) (-28.6097, -65.7179) (-28.1214, -65.9001) (-27.6326, -66.0792) (-27.1433, -66.2551) (-26.6534, -66.4278) (-26.163, -66.5974) (-25.6721, -66.7638) (-25.1806, -66.927) (-24.6885, -67.0871) (-24.1958, -67.244) (-23.7026, -67.3978) (-23.2087, -67.5484) (-22.7144, -67.6958) (-22.2194, -67.8401) (-21.7238, -67.9811) (-21.2277, -68.1191) (-20.7311, -68.2538) (-20.2338, -68.3854) (-19.736, -68.5137) (-19.2377, -68.6389) (-18.7388, -68.7609) (-18.2393, -68.8798) (-17.7394, -68.9954) (-17.2389, -69.1078) (-16.7379, -69.217) (-16.2363, -69.323) (-15.7343, -69.4258) (-15.2318, -69.5254) (-14.7289, -69.6218) (-14.2255, -69.7149) (-13.7216, -69.8049) (-13.2173, -69.8915) (-12.7125, -69.975) (-12.2074, -70.0552) (-11.7018, -70.1322) (-11.1959, -70.2059) (-10.6896, -70.2764) (-10.1829, -70.3436) (-9.6759, -70.4075) (-9.1686, -70.4683) (-8.661, -70.5257) (-8.1531, -70.5799) (-7.6449, -70.6308) (-7.1364, -70.6784) (-6.6277, -70.7228) (-6.1188, -70.7639) (-5.6096, -70.8017) (-5.1003, -70.8362) (-4.5907, -70.8674) (-4.0811, -70.8954) (-3.5712, -70.9201) (-3.0613, -70.9415) (-2.5513, -70.9596) (-2.0411, -70.9744) (-1.5309, -70.9859) (-1.0206, -70.9941) (-0.5103, -70.9991) (0, -71.0007) (0.5103, -70.9991) (1.0206, -70.9941) (1.5309, -70.9859) (2.0411, -70.9744) (2.5512, -70.9596) (3.0613, -70.9415) (3.5712, -70.9201) (4.0811, -70.8954) (4.5907, -70.8674) (5.1002, -70.8362) (5.6096, -70.8017) (6.1187, -70.7639) (6.6276, -70.7228) (7.1363, -70.6784) (7.6447, -70.6308) (8.1529, -70.5799) (8.6608, -70.5257) (9.1683, -70.4683) (9.6756, -70.4076) (10.1825, -70.3436) (10.6891, -70.2764) (11.1953, -70.2059) (11.7011, -70.1322) (12.2065, -70.0553) (12.7115, -69.9751) (13.2161, -69.8917) (13.7202, -69.805) (14.2238, -69.7151) (14.727, -69.622) (15.2297, -69.5257) (15.7318, -69.4261) (16.2335, -69.3234) (16.7346, -69.2175) (17.2352, -69.1083) (17.7352, -68.996) (18.2346, -68.8805) (18.7335, -68.7617) (19.2317, -68.6399) (19.7293, -68.5148) (20.2264, -68.3866) (20.7227, -68.2552) (21.2185, -68.1207) (21.7136, -67.983) (22.208, -67.8421) (22.7018, -67.6981) (23.1948, -67.551) (23.6872, -67.4008) (24.1789, -67.2474) (24.6699, -67.0909) (25.1602, -66.9313) (25.6497, -66.7686) (26.1386, -66.6028) (26.6267, -66.4339) (27.1141, -66.2618) (27.6008, -66.0867) (28.0867, -65.9085) (28.5719, -65.7272) (29.0563, -65.5428) (29.54, -65.3554) (30.023, -65.1648) (30.5052, -64.9712) (30.9867, -64.7745) (31.4674, -64.5748) (31.9475, -64.3719) (32.4267, -64.166) (32.9053, -63.9571) (33.3831, -63.745) (33.8603, -63.5299) (34.3367, -63.3117) (34.8124, -63.0904) (35.2875, -62.8661) (35.7619, -62.6386) (36.2356, -62.4081) (36.7086, -62.1745) (37.181, -61.9378) (37.6528, -61.698) (38.124, -61.455) (38.5946, -61.209) (39.0646, -60.9598) (39.5341, -60.7075) (40.003, -60.452) (40.4714, -60.1934) (40.9394, -59.9316) (41.4069, -59.6666) (41.8739, -59.3984) (42.3406, -59.127) (42.8069, -58.8523) (43.4481, -58.4698) (43.9715, -58.1517) (44.3779, -57.9011) (44.6679, -57.7205) knots 0 0 0 0 0 0.014541 0.020333 0.02611 0.031872 0.03762 0.043355 0.049078 0.054789 0.060489 0.066178 0.071857 0.077527 0.083187 0.088839 0.094483 0.10012 0.105749 0.111371 0.116986 0.122595 0.128199 0.133797 0.139389 0.144976 0.150559 0.156136 0.16171 0.167279 0.172845 0.178407 0.183965 0.18952 0.195072 0.20062 0.206166 0.211709 0.21725 0.222788 0.228323 0.233857 0.239388 0.244918 0.250445 0.255971 0.261495 0.267017 0.272538 0.278057 0.283575 0.289092 0.294608 0.300122 0.305635 0.311147 0.316658 0.322169 0.327678 0.333186 0.338694 0.344201 0.349707 0.355213 0.360718 0.366222 0.371726 0.377229 0.382732 0.388235 0.393737 0.399238 0.404739 0.41024 0.415741 0.421241 0.426741 0.432241 0.43774 0.44324 0.448739 0.454238 0.459737 0.465236 0.470734 0.476233 0.481731 0.48723 0.492728 0.498227 0.503725 0.509224 0.514722 0.520221 0.525719 0.531218 0.536717 0.542216 0.547715 0.553214 0.558714 0.564214 0.569713 0.575214 0.580714 0.586215 0.591716 0.597217 0.602718 0.60822 0.613723 0.619225 0.624728 0.630232 0.635736 0.641241 0.646746 0.652251 0.657758 0.663264 0.668772 0.67428 0.679789 0.685299 0.690809 0.69632 0.701832 0.707345 0.712859 0.718374 0.72389 0.729407 0.734925 0.740444 0.745965 0.751487 0.75701 0.762535 0.768061 0.773588 0.779117 0.784648 0.790181 0.795715 0.801252 0.80679 0.812331 0.817873 0.823418 0.828965 0.834515 0.840067 0.845622 0.85118 0.85674 0.862304 0.867871 0.873441 0.879014 0.884591 0.890172 0.895757 0.901345 0.906938 0.912535 0.918137 0.923743 0.929355 0.934971 0.940593 0.946221 0.951854 0.957493 0.963139 0.968791 0.974449 0.980115 0.985788 1 1 1 1 1
  line L7 (44.6679, -57.7205) -> (47.1325, -53.2266)
  arc A15 (4.5969, -37.0887) -> (23.8174, -61.1986) centre (28.8377, -37.4801) ccw
  spline S1 degree 3 poles (23.923, -63.1268) (24.0467, -63.086) (24.1612, -63.0216) (24.3592, -62.8523) (24.4407, -62.7492) (24.5595, -62.5175) (24.5958, -62.3911) (24.6178, -62.1316) (24.6033, -62.0009) (24.5251, -61.7525) (24.4622, -61.6371) (24.3075, -61.4513) (24.2222, -61.3781) (24.0311, -61.2629) (23.9266, -61.2217) (23.8174, -61.1986) knots 0 0 0 0 0.148947 0.148947 0.297893 0.297893 0.44684 0.44684 0.595787 0.595787 0.744733 0.744733 0.872367 0.872367 1 1 1 1
  spline S2 degree 3 poles (23.923, -63.1268) (23.6264, -63.2244) (21.6991, -63.8462) (18.9298, -64.6237) (14.7719, -65.5721) (11.4157, -66.1631) (7.1944, -66.6887) (3.8013, -66.9375) (-0.4475, -67.0324) (-3.8473, -66.9351) (-8.0854, -66.5978) (-11.4616, -66.156) (-15.6527, -65.3916) (-18.978, -64.6118) (-23.0925, -63.431) (-25.7434, -62.5289) (-27.5645, -61.8359) (-27.7718, -61.756) knots -0.770978 -0.770978 -0.770978 -0.770978 -0.760435 -0.70257 -0.673637 -0.615772 -0.58684 -0.528974 -0.500042 -0.442177 -0.413244 -0.355379 -0.326446 -0.268581 -0.239649 -0.181783 -0.174342 -0.174342 -0.174342 -0.174342
  spline S3 degree 3 poles (-27.5161, -59.8282) (-27.6456, -59.8417) (-27.7712, -59.8804) (-28.0006, -60.0037) (-28.1022, -60.0872) (-28.2675, -60.2884) (-28.3298, -60.4042) (-28.4064, -60.6531) (-28.42, -60.7838) (-28.3964, -61.0432) (-28.3594, -61.1693) (-28.2435, -61.3919) (-28.1687, -61.4881) (-27.9885, -61.6491) (-27.8845, -61.7126) (-27.7718, -61.756) knots 0 0 0 0 0.145866 0.145866 0.291731 0.291731 0.437597 0.437597 0.583462 0.583462 0.729328 0.729328 0.864664 0.864664 1 1 1 1
  arc A16 (-27.5161, -59.8282) -> (-20.671, -58.4236) centre (-31.2017, -24.4856) ccw
  arc A17 (-20.671, -58.4236) -> (-4.7434, -37.0245) centre (-27.3796, -36.8033) ccw
  arc A18 (-3.4858, -36.0681) -> (-4.7434, -37.0245) centre (-3.7435, -37.0343) ccw
  arc A19 (-3.4858, -36.0681) -> (3.3494, -36.1037) centre (0, -23) ccw
  arc A20 (4.5969, -37.0887) -> (3.3494, -36.1037) centre (3.597, -37.0726) ccw
  circle A21 centre (0, -23) radius 8.525
  arc A22 (11.9265, -19.1744) -> (-5.0879, -11.555) centre (0, -23) ccw
  line L8 (-4.9441, 2.4403) -> (-9.0832, -7.6778)
  dimension "d31" = 2
  dimension "d33" = 2
  constraints: 18 centre point, 8 point on circle, 5 end point, 3 tangent, 1 coincident, 1 parallel, 1 point on line, 10 other
  measures "d31" diameter of A5
  measures "d33" radial gap between concentric circles of A2 A6
chamfer "面取り1" distance 1.75 angle 45 2 edges at (-7.8066, -8.8137, 0) (-1.5, 0, 0)
sketch "スケッチ8" plane through (0, 0, 5) normal (0, 0, 1) x (1, 0, 0)
  arc A0 (47.1325, -53.2266) -> (45.758, -51.8784) centre (46.2557, -52.7457) ccw projected
  arc A1 (33.009, -56.7784) -> (45.758, -51.8784) centre (23.6069, -13.28) ccw projected
  arc A2 (11.1932, -28.6204) -> (33.009, -56.7784) centre (28.8377, -37.4801) ccw projected
  arc A3 (11.1932, -28.6204) -> (-5.0879, -11.555) centre (0, -23) ccw projected
  arc A4 (-9.0832, -7.6778) -> (-5.0879, -11.555) centre (-6.3066, -8.8137) ccw projected
  line L0 (-9.0832, -7.6778) -> (-4.9441, 2.4403) projected
  line L1 (-4.9441, 2.4403) -> (-10.1922, -6.5439) projected
  arc A5 (-10.1922, -6.5439) -> (-10.7715, -8.253) centre (-6.3066, -8.8137) ccw projected
  line L2 (-10.7715, -8.253) -> (-12.4274, -21.4394) projected
  arc A6 (-12.4274, -21.4394) -> (-11.1841, -28.6384) centre (0, -23) ccw projected
  arc A7 (-22.0046, -54.1258) -> (-11.1841, -28.6384) centre (-27.3796, -36.8033) ccw projected
  arc A8 (-45.6895, -51.9306) -> (-22.0046, -54.1258) centre (-31.2017, -24.4856) ccw projected
  arc A9 (-45.6895, -51.9306) -> (-47.014, -53.3291) centre (-46.1563, -52.815) ccw projected
  line L3 (-47.014, -53.3291) -> (-44.145, -58.1151) projected
  line L4 (44.6679, -57.7205) -> (47.1325, -53.2266) projected
  arc A10 (4.5969, -37.0887) -> (23.8174, -61.1986) centre (28.8377, -37.4801) ccw projected
  arc A11 (-27.5161, -59.8282) -> (-20.671, -58.4236) centre (-31.2017, -24.4856) ccw projected
  arc A12 (-20.671, -58.4236) -> (-4.7434, -37.0245) centre (-27.3796, -36.8033) ccw projected
  arc A13 (-3.4858, -36.0681) -> (-4.7434, -37.0245) centre (-3.7435, -37.0343) ccw projected
  arc A14 (-3.4858, -36.0681) -> (3.3494, -36.1037) centre (0, -23) ccw projected
  arc A15 (4.5969, -37.0887) -> (3.3494, -36.1037) centre (3.597, -37.0726) ccw projected
  circle A16 centre (0, -23) radius 8.525 projected
  line L5 (-4.9441, 2.4403) -> (-9.0832, -7.6778) projected
  arc A17 (-9.0832, -7.6778) -> (-5.0879, -11.555) centre (-6.3066, -8.8137) ccw projected
  arc A18 (11.9265, -19.1744) -> (-5.0879, -11.555) centre (0, -23) ccw projected
  line L6 (5.2372, 1.6799) -> (11.9265, -19.1744) projected
  arc A19 (5.2372, 1.6799) -> (-4.7491, 2.7742) centre (0, 0) ccw projected
  line L7 (-4.7491, 2.7742) -> (-4.9441, 2.4403) projected
  circle A20 centre (-6.3066, -8.8137) radius 1.5 projected
  circle A21 centre (0, 0) radius 1.5 projected
  arc A22 (7.246, 1.9652) -> (-4.9441, 2.4403) centre (1.0644, -0.0177) ccw
  line L8 (7.246, 1.9652) -> (13.8309, -18.5636)
  line L9 (11.9265, -19.1744) -> (5.2372, 1.6799) projected
  arc A23 (11.9265, -19.1744) -> (13.8309, -18.5636) centre (12.8787, -18.869) ccw
  arc A24 (11.1932, -28.6204) -> (-5.0879, -11.555) centre (0, -23) ccw projected
  arc A25 (47.1325, -53.2266) -> (45.758, -51.8784) centre (46.2557, -52.7457) ccw projected
  line L10 (44.6679, -57.7205) -> (47.1325, -53.2266) projected
  spline S0 degree 4 poles (-44.145, -58.1151) (-43.8381, -58.3003) (-43.4088, -58.5568) (-42.8575, -58.8816) (-42.1841, -59.2711) (-41.6963, -59.5497) (-41.2094, -59.8243) (-40.7232, -60.0949) (-40.2377, -60.3617) (-39.7528, -60.6247) (-39.2684, -60.8839) (-38.7844, -61.1395) (-38.3007, -61.3914) (-37.8172, -61.6398) (-37.334, -61.8846) (-36.8508, -62.1259) (-36.3678, -62.3637) (-35.8847, -62.5981) (-35.4015, -62.8291) (-34.9183, -63.0567) (-34.4349, -63.281) (-33.9513, -63.502) (-33.4675, -63.7196) (-32.9834, -63.934) (-32.499, -64.1451) (-32.0143, -64.3529) (-31.5292, -64.5576) (-31.0437, -64.7589) (-30.5578, -64.9571) (-30.0715, -65.1521) (-29.5847, -65.3439) (-29.0974, -65.5325) (-28.6097, -65.7179) (-28.1214, -65.9001) (-27.6326, -66.0792) (-27.1433, -66.2551) (-26.6534, -66.4278) (-26.163, -66.5974) (-25.6721, -66.7638) (-25.1806, -66.927) (-24.6885, -67.0871) (-24.1958, -67.244) (-23.7026, -67.3978) (-23.2087, -67.5484) (-22.7144, -67.6958) (-22.2194, -67.8401) (-21.7238, -67.9811) (-21.2277, -68.1191) (-20.7311, -68.2538) (-20.2338, -68.3854) (-19.736, -68.5137) (-19.2377, -68.6389) (-18.7388, -68.7609) (-18.2393, -68.8798) (-17.7394, -68.9954) (-17.2389, -69.1078) (-16.7379, -69.217) (-16.2363, -69.323) (-15.7343, -69.4258) (-15.2318, -69.5254) (-14.7289, -69.6218) (-14.2255, -69.7149) (-13.7216, -69.8049) (-13.2173, -69.8915) (-12.7125, -69.975) (-12.2074, -70.0552) (-11.7018, -70.1322) (-11.1959, -70.2059) (-10.6896, -70.2764) (-10.1829, -70.3436) (-9.6759, -70.4075) (-9.1686, -70.4683) (-8.661, -70.5257) (-8.1531, -70.5799) (-7.6449, -70.6308) (-7.1364, -70.6784) (-6.6277, -70.7228) (-6.1188, -70.7639) (-5.6096, -70.8017) (-5.1003, -70.8362) (-4.5907, -70.8674) (-4.0811, -70.8954) (-3.5712, -70.9201) (-3.0613, -70.9415) (-2.5513, -70.9596) (-2.0411, -70.9744) (-1.5309, -70.9859) (-1.0206, -70.9941) (-0.5103, -70.9991) (0, -71.0007) (0.5103, -70.9991) (1.0206, -70.9941) (1.5309, -70.9859) (2.0411, -70.9744) (2.5512, -70.9596) (3.0613, -70.9415) (3.5712, -70.9201) (4.0811, -70.8954) (4.5907, -70.8674) (5.1002, -70.8362) (5.6096, -70.8017) (6.1187, -70.7639) (6.6276, -70.7228) (7.1363, -70.6784) (7.6447, -70.6308) (8.1529, -70.5799) (8.6608, -70.5257) (9.1683, -70.4683) (9.6756, -70.4076) (10.1825, -70.3436) (10.6891, -70.2764) (11.1953, -70.2059) (11.7011, -70.1322) (12.2065, -70.0553) (12.7115, -69.9751) (13.2161, -69.8917) (13.7202, -69.805) (14.2238, -69.7151) (14.727, -69.622) (15.2297, -69.5257) (15.7318, -69.4261) (16.2335, -69.3234) (16.7346, -69.2175) (17.2352, -69.1083) (17.7352, -68.996) (18.2346, -68.8805) (18.7335, -68.7617) (19.2317, -68.6399) (19.7293, -68.5148) (20.2264, -68.3866) (20.7227, -68.2552) (21.2185, -68.1207) (21.7136, -67.983) (22.208, -67.8421) (22.7018, -67.6981) (23.1948, -67.551) (23.6872, -67.4008) (24.1789, -67.2474) (24.6699, -67.0909) (25.1602, -66.9313) (25.6497, -66.7686) (26.1386, -66.6028) (26.6267, -66.4339) (27.1141, -66.2618) (27.6008, -66.0867) (28.0867, -65.9085) (28.5719, -65.7272) (29.0563, -65.5428) (29.54, -65.3554) (30.023, -65.1648) (30.5052, -64.9712) (30.9867, -64.7745) (31.4674, -64.5748) (31.9475, -64.3719) (32.4267, -64.166) (32.9053, -63.9571) (33.3831, -63.745) (33.8603, -63.5299) (34.3367, -63.3117) (34.8124, -63.0904) (35.2875, -62.8661) (35.7619, -62.6386) (36.2356, -62.4081) (36.7086, -62.1745) (37.181, -61.9378) (37.6528, -61.698) (38.124, -61.455) (38.5946, -61.209) (39.0646, -60.9598) (39.5341, -60.7075) (40.003, -60.452) (40.4714, -60.1934) (40.9394, -59.9316) (41.4069, -59.6666) (41.8739, -59.3984) (42.3406, -59.127) (42.8069, -58.8523) (43.4481, -58.4698) (43.9715, -58.1517) (44.3779, -57.9011) (44.6679, -57.7205) knots 0 0 0 0 0 0.014541 0.020333 0.02611 0.031872 0.03762 0.043355 0.049078 0.054789 0.060489 0.066178 0.071857 0.077527 0.083187 0.088839 0.094483 0.10012 0.105749 0.111371 0.116986 0.122595 0.128199 0.133797 0.139389 0.144976 0.150559 0.156136 0.16171 0.167279 0.172845 0.178407 0.183965 0.18952 0.195072 0.20062 0.206166 0.211709 0.21725 0.222788 0.228323 0.233857 0.239388 0.244918 0.250445 0.255971 0.261495 0.267017 0.272538 0.278057 0.283575 0.289092 0.294608 0.300122 0.305635 0.311147 0.316658 0.322169 0.327678 0.333186 0.338694 0.344201 0.349707 0.355213 0.360718 0.366222 0.371726 0.377229 0.382732 0.388235 0.393737 0.399238 0.404739 0.41024 0.415741 0.421241 0.426741 0.432241 0.43774 0.44324 0.448739 0.454238 0.459737 0.465236 0.470734 0.476233 0.481731 0.48723 0.492728 0.498227 0.503725 0.509224 0.514722 0.520221 0.525719 0.531218 0.536717 0.542216 0.547715 0.553214 0.558714 0.564214 0.569713 0.575214 0.580714 0.586215 0.591716 0.597217 0.602718 0.60822 0.613723 0.619225 0.624728 0.630232 0.635736 0.641241 0.646746 0.652251 0.657758 0.663264 0.668772 0.67428 0.679789 0.685299 0.690809 0.69632 0.701832 0.707345 0.712859 0.718374 0.72389 0.729407 0.734925 0.740444 0.745965 0.751487 0.75701 0.762535 0.768061 0.773588 0.779117 0.784648 0.790181 0.795715 0.801252 0.80679 0.812331 0.817873 0.823418 0.828965 0.834515 0.840067 0.845622 0.85118 0.85674 0.862304 0.867871 0.873441 0.879014 0.884591 0.890172 0.895757 0.901345 0.906938 0.912535 0.918137 0.923743 0.929355 0.934971 0.940593 0.946221 0.951854 0.957493 0.963139 0.968791 0.974449 0.980115 0.985788 1 1 1 1 1 projected
  line L11 (-47.014, -53.3291) -> (-44.145, -58.1151) projected
  arc A26 (-45.6895, -51.9306) -> (-47.014, -53.3291) centre (-46.1563, -52.815) ccw projected
  arc A27 (-22.0046, -54.1258) -> (-45.6895, -51.9306) centre (-31.2017, -24.4856) ccw projected
  arc A28 (-11.1841, -28.6384) -> (-22.0046, -54.1258) centre (-27.3796, -36.8033) ccw projected
  arc A29 (-12.4274, -21.4394) -> (-11.1841, -28.6384) centre (0, -23) ccw projected
  line L12 (-12.4274, -21.4394) -> (-10.7715, -8.253) projected
  arc A30 (-10.7715, -8.253) -> (-10.1922, -6.5439) centre (-6.3066, -8.8137) ccw projected
  line L13 (-10.1922, -6.5439) -> (-4.7491, 2.7742) projected
  arc A31 (5.2372, 1.6799) -> (-4.7491, 2.7742) centre (0, 0) ccw projected
  line L14 (11.9265, -19.1744) -> (5.2372, 1.6799) projected
  arc A32 (11.1932, -28.6204) -> (11.9265, -19.1744) centre (0, -23) ccw projected
  arc A33 (33.009, -56.7784) -> (11.1932, -28.6204) centre (28.8377, -37.4801) ccw projected
  arc A34 (45.758, -51.8784) -> (33.009, -56.7784) centre (23.6069, -13.28) ccw projected
  circle A35 centre (0, -23) radius 8.525 projected
  dimension "d37" = 2
  constraints: 13 centre point, 4 point on circle, 4 tangent, 2 end point, 1 parallel, 6 other
  measures "d37" distance between parallel lines of L6 L8
